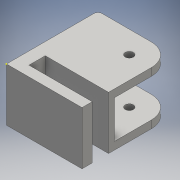
# Autodesk Inventor part: Maintients poullies V3 Beta
Saved by Autodesk Inventor 2016 (Build 200138000, 138)
## iProperties
Created: 2016-02-24
Part Number: Maintients poullies V3 Beta
Material: Generic
Document SubType Name: Modeling
Designer: Thetheos
Density: 1 g/cm^3
Appearance: Default
Author: Thetheos
Autodesk Inventor part; units mm, degrees
ref_plane "YZ Plane" through (0, 0, 0) normal (1, 0, 0) x (0, 1, 0)
ref_plane "XZ Plane" through (0, 0, 0) normal (0, 1, 0) x (-1, 0, 0)
ref_plane "XY Plane" through (0, 0, 0) normal (0, 0, 1) x (1, 0, 0)
sketch "Sketch1" plane through (0, 0, 0) normal (0, 0, 1) x (1, 0, 0)
  line L0 (6, 5) -> (6, 13)
  line L1 (0, 16) -> (0, 0)
  arc A0 (37.0043, 34) -> (18.539, 41.6832) centre (26.1732, 34) ccw
  line L2 (18.539, 41.6832) -> (0, 16)
  circle A1 centre (26.1732, 34) radius 2
  line L3 (37.0043, 5) -> (37.0043, 0)
  line L4 (6, 5) -> (37.0043, 5)
  line L5 (0, 0) -> (37.0043, 0)
  line L6 (6, 13) -> (37.0043, 13)
  line L7 (0, 16) -> (37.0043, 16)
  line L8 (37.0043, 34) -> (37.0043, 13)
  dimension "d3" = 8
  dimension "d6" = 18
  dimension "d7" = 20
  dimension "d8" = 4
  dimension "d9" = 3
  dimension "d10" = 5
  dimension "d11" = 16
  dimension "d12" = 37.0043
  dimension "d13" = 31.0043
  constraints: 18 end point, 2 centre point, 2 point on circle, 1 coincident, 1 horizontal
  measures "d3" distance of L0.start L0.end
  measures "d6" distance of L7.end L8.start
  measures "d7" distance of L8.start L2.start
  measures "d8" diameter of A1
  measures "d9" distance between parallel lines of L6 L7
  measures "d10" distance between parallel lines of L5 L4
  measures "d11" distance between parallel lines of L5 L7
  measures "d12" distance between parallel lines of L8 L1
  measures "d13" distance between parallel lines of L8 L0
extrude "Extrusion1" add sketch "Sketch1" along normal blind 26
sketch "Sketch2" plane through (0, 0, 26) normal (0, 0, 1) x (1, 0, 0)
  point P0 (0, 0)
sketch "Sketch3" plane through (37.0043, 13, 0) normal (1, 0, 0) x (0, 0, -1)
  line L0 (0, 0) -> (-26, 0) projected
  line L1 (-13, 38) -> (-3.75, 38)
  line L2 (-3.75, 38) -> (-3.75, 3)
  line L3 (-13, 38) -> (-22.25, 38)
  line L4 (-22.25, 38) -> (-22.25, 3)
  line L5 (-22.25, 3) -> (-3.75, 3)
  line L6 (0, 0) -> (-26, 0) projected
  point P0 (0, -13)
  point P1 (-26, 3)
  dimension "d19" = 9.25
  dimension "d20" = 9.25
  constraints: 10 end point, 1 horizontal, 1 parallel
  measures "d19" distance of L1.start L1.end
  measures "d20" distance of L1.start L3.end
extrude "Extrusion2" cut sketch "Sketch3" against normal through all
sketch "Sketch4" plane through (0, 0, 26) normal (0, 0, 1) x (1, 0, 0)
  arc A0 (37.0043, 34) -> (18.539, 41.6832) centre (26.1732, 34) ccw projected
  line L0 (26.1732, 44.8311) -> (0, 44.8311)
  line L1 (18.539, 41.6832) -> (0, 16) projected
  line L2 (0, 44.8311) -> (0, 16)
  point P0 (0, 0)
  constraints: 4 end point, 1 horizontal, 1 perpendicular, 1 point on circle, 1 tangent
extrude "Extrusion3" add sketch "Sketch4" against normal blind 26
sketch "Sketch5" plane through (37.0043, 13, 0) normal (1, 0, 0) x (0, 0, -1)
  line L0 (-22.25, 3) -> (-22.25, 21) projected
  line L1 (-22.25, 3) -> (-3.75, 3)
  line L2 (-3.75, 3) -> (-3.75, 33)
  line L3 (-3.75, 33) -> (-22.25, 33)
  line L4 (-22.25, 33) -> (-22.25, 3)
  point P0 (0, -13)
  constraints: 8 end point, 2 parallel, 1 horizontal, 1 perpendicular
extrude "Extrusion4" cut sketch "Sketch5" against normal through all
fillet "Fillet1" radius 2 1 edges at (0, 44.8311, 1.875)
fillet "Fillet2" radius 2 1 edges at (0, 44.8311, 24.125)
body "Solid1"
